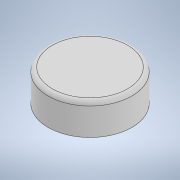
# Autodesk Inventor part: knob_top
Saved by Autodesk Inventor 2022 (Build 260153000, 153)
## iProperties
Created: 2022-06-07
Part Number: knob_top
Material: Generic
Document SubType Name: Modeling
Designer: Jacob
Density: 1 g/cm^3
Appearance: Default
Author: Jacob
Autodesk Inventor part; units mm, degrees
ref_plane "YZ Plane" through (0, 0, 0) normal (1, 0, 0) x (0, 1, 0)
ref_plane "XZ Plane" through (0, 0, 0) normal (0, 1, 0) x (-1, 0, 0)
ref_plane "XY Plane" through (0, 0, 0) normal (0, 0, 1) x (1, 0, 0)
sketch "Sketch1" plane through (0, 0, 0) normal (0, 1, 0) x (-1, 0, 0)
  circle A0 centre (0, 0) radius 2.3
  circle A1 centre (0, 0) radius 10
  circle A2 centre (0, 0) radius 2.1
  dimension "d0" = 0.2
  constraints: 3 centre point, 6 other
  measures "d0" radial gap between concentric circles of A0 A2
extrude "Extrusion1" add sketch "Sketch1" along normal blind 7.5 contours A0 | A1 | A2
fillet "Fillet1" radius 1 1 edges at (10, 7.5, 0)
extrude "Extrusion2" add sketch "Sketch1" against normal blind 2 contours A2
chamfer "Chamfer1" distance 0.5 angle 45 1 edges at (2.1, -2, 0)
body "Solid1"
